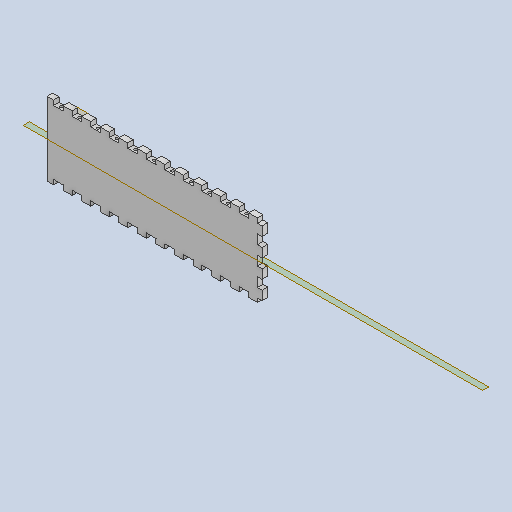
# Autodesk Inventor part: 00_Baseplate_Simmo_side3
Saved by Autodesk Inventor 2022 (Build 260153000, 153)
## iProperties
Created: 2022-04-28
Part Number: 00_Baseplate_Simmo_side3
Material: Generisch
Document SubType Name: Modeling
Designer: diederichbenedict
Density: 1 g/cm^3
Appearance: Vorgabe
Author: diederichbenedict
Autodesk Inventor part; units mm, degrees
ref_plane "YZ Plane" through (0, 0, 0) normal (1, 0, 0) x (0, 1, 0)
ref_plane "XZ Plane" through (0, 0, 0) normal (0, 1, 0) x (-1, 0, 0)
ref_plane "XY Plane" through (0, 0, 0) normal (0, 0, 1) x (1, 0, 0)
ref_plane "Arbeitsebene1" through (0, 0, 0) normal (0, 0, 1) x (1, 0, 0)
sketch "Skizze1" plane through (0, 0, 0) normal (0, 0, 1) x (1, 0, 0)
  line L0 (0, 5) -> (10, 5)
  line L1 (10, 0) -> (0, 0)
  line L2 (10, 0) -> (10, 5)
  line L3 (442.7944, 5) -> (442.7944, 0)
  line L4 (0, -68) -> (10, -68)
  line L5 (0, 5) -> (229.5237, 5)
  line L6 (229.5237, 5) -> (229.5237, -68)
  line L7 (229.5237, -68) -> (0, -68)
  line L8 (0, -68) -> (0, 5)
  line L9 (0, -68) -> (229.5237, -68)
  line L10 (229.5237, -68) -> (229.5237, -74)
  line L11 (229.5237, -74) -> (0, -74)
  line L12 (0, -74) -> (0, -68)
  line L13 (0, 0) -> (0, 5)
  line L14 (238.603, -69) -> (238.603, -74)
  line L15 (230.1, -69) -> (230.1, -74)
  line L16 (230.1, -74) -> (220.1, -74)
  line L17 (229.5237, 0.1) -> (229.5237, 5)
  point P0 (450, -68)
  point P1 (450, 0)
  point P2 (442.7944, 5)
  point P3 (450, -68)
extrude "Extrusion1" add sketch "Skizze1" along normal blind 6
sketch "Skizze2" plane through (0, 0, 0) normal (0, 0, -1) x (1, 0, 0)
  line L0 (20, 0) -> (20, -5) projected
  line L1 (10, -5) -> (10, 0) projected
  line L2 (0, -5) -> (0, 74) projected
  line L3 (9.8, -5) -> (20.2, -5)
  line L4 (20.2, -5) -> (20.2, 0)
  line L5 (20.2, 0) -> (9.8, 0)
  line L6 (9.8, 0) -> (9.8, -5)
  point P0 (0, 0)
  dimension "d6" = 0
  dimension "d17" = 0.2
  dimension "d18" = 0.2
  constraints: 8 end point, 2 parallel, 1 horizontal, 1 perpendicular
  measures "d6" distance from line of L1.end L5
  measures "d17" distance between parallel lines of L4 L0
  measures "d18" distance between parallel lines of L6 L1
extrude "Extrusion2" cut sketch "Skizze2" against normal blind 6
sketch "Skizze3" plane through (20.2, 5, 0) normal (0, 1, 0) x (1, 0, 0)
  line L0 (209.3237, 0) -> (0, 0) projected
  line L1 (-10.4, -6) -> (0, -6) projected
  line L2 (0, 0) -> (0, -6) projected
  circle A0 centre (-5.2, -3) radius 1.5
  line L3 (-10.4, -6) -> (-10.4, 0) projected
  point P0 (-20.2, 0)
  point P1 (4.8, 3)
  point P2 (429.8, 0)
  point P3 (429.8, -6)
  dimension "d16" = 3
  dimension "d19" = 5.2
  constraints: 1 centre point
  measures "d16" diameter of A0
  measures "d19" distance from line of A0.centre L3
hole "Bohrung1" at (15, 5, 3) direction (0, -1, 0) diameter 3 depth 20
pattern_linear "Rechteckige Anordnung1" count 24 spacing 20 along (1, 0, 0) of "Extrusion2", "Bohrung1"
ref_plane "Arbeitsebene2" through (0, -34.5, 0) normal (0, -1, 0) x (1, 0, 0)
mirror "Spiegeln1" about plane through (0, -34.5, 0) normal (0, -1, 0) of "Extrusion2", "Bohrung1", "Rechteckige Anordnung1"
sketch "Skizze4" plane through (0, 5, 6) normal (0, 1, 0) x (1, 0, 0)
  line L0 (9.8356, 19.8689) -> (14.6897, 16.3421) projected
  line L1 (20.45, 24.2705) -> (14.6897, 16.3421) projected
  line L2 (15.5959, 27.7972) -> (20.45, 24.2705) projected
  line L3 (15.5959, 27.7972) -> (9.8356, 19.8689) projected
  line L4 (9.8, 0) -> (0, 0) projected
  line L5 (3, 0) -> (-2.0103, 0)
  line L6 (-2.0103, 0) -> (-2.0103, 6)
  line L7 (-2.0103, 6) -> (3, 6)
  line L8 (3, 6) -> (3, 0)
  line L9 (0, 6) -> (0, 0) projected
  line L10 (2.8165, 0) -> (2.8165, 6)
  point P0 (-2.0103, 2.2794)
  point P1 (0, 6)
  point P2 (0, 0)
  point P3 (0, 0)
  dimension "d25" = 3
  constraints: 10 end point, 2 parallel, 1 horizontal, 1 perpendicular, 1 point on line, 1 vertical, 3 other
  measures "d25" distance between parallel lines of L9 L8
extrude "Extrusion3" cut sketch "Skizze4" against normal through all contours L3 L2 L1 L0 | L4 L9 L7 L10 | L5 L6 L7 L9
sketch "Skizze5" plane through (0, 0, 6) normal (0, 0, 1) x (1, 0, 0)
  line L0 (2.8165, 5) -> (2.8165, -74) projected
  line L1 (2.8165, -74) -> (9.8, -74) projected
  line L2 (9.8, -74) -> (9.8, -69) projected
  line L3 (9.8, -69) -> (20.2, -69) projected
  line L4 (20.2, -69) -> (20.2, -74) projected
  line L5 (20.2, -74) -> (29.8, -74) projected
  line L6 (29.8, -74) -> (29.8, -69) projected
  line L7 (29.8, -69) -> (40.2, -69) projected
  line L8 (40.2, -69) -> (40.2, -74) projected
  line L9 (40.2, -74) -> (49.8, -74) projected
  line L10 (49.8, -74) -> (49.8, -69) projected
  line L11 (49.8, -69) -> (60.2, -69) projected
  line L12 (60.2, -69) -> (60.2, -74) projected
  line L13 (60.2, -74) -> (69.8, -74) projected
  line L14 (69.8, -74) -> (69.8, -69) projected
  line L15 (69.8, -69) -> (80.2, -69) projected
  line L16 (80.2, -69) -> (80.2, -74) projected
  line L17 (80.2, -74) -> (89.8, -74) projected
  line L18 (89.8, -74) -> (89.8, -69) projected
  line L19 (89.8, -69) -> (100.2, -69) projected
  line L20 (100.2, -69) -> (100.2, -74) projected
  line L21 (100.2, -74) -> (109.8, -74) projected
  line L22 (109.8, -74) -> (109.8, -69) projected
  line L23 (109.8, -69) -> (120.2, -69) projected
  line L24 (120.2, -69) -> (120.2, -74) projected
  line L25 (120.2, -74) -> (129.8, -74) projected
  line L26 (129.8, -74) -> (129.8, -69) projected
  line L27 (129.8, -69) -> (140.2, -69) projected
  line L28 (140.2, -69) -> (140.2, -74) projected
  line L29 (140.2, -74) -> (149.8, -74) projected
  line L30 (149.8, -74) -> (149.8, -69) projected
  line L31 (149.8, -69) -> (160.2, -69) projected
  line L32 (160.2, -69) -> (160.2, -74) projected
  line L33 (160.2, -74) -> (169.8, -74) projected
  line L34 (169.8, -74) -> (169.8, -69) projected
  line L35 (169.8, -69) -> (180.2, -69) projected
  line L36 (180.2, -69) -> (180.2, -74) projected
  line L37 (180.2, -74) -> (189.8, -74) projected
  line L38 (189.8, -74) -> (189.8, -69) projected
  line L39 (189.8, -69) -> (200.2, -69) projected
  line L40 (200.2, -69) -> (200.2, -74) projected
  line L41 (200.2, -74) -> (209.8, -74) projected
  line L42 (209.8, -74) -> (209.8, -69) projected
  line L43 (209.8, -69) -> (220.2, -69) projected
  line L44 (220.2, -69) -> (220.2, -74) projected
  line L45 (220.2, -74) -> (229.5237, -74) projected
  line L46 (229.5237, -74) -> (229.5237, 5) projected
  line L47 (229.5237, 5) -> (220.2, 5) projected
  line L48 (220.2, 5) -> (220.2, 0) projected
  line L49 (220.2, 0) -> (209.8, 0) projected
  line L50 (209.8, 0) -> (209.8, 5) projected
  line L51 (209.8, 5) -> (200.2, 5) projected
  line L52 (200.2, 5) -> (200.2, 0) projected
  line L53 (200.2, 0) -> (189.8, 0) projected
  line L54 (189.8, 0) -> (189.8, 5) projected
  line L55 (189.8, 5) -> (180.2, 5) projected
  line L56 (180.2, 5) -> (180.2, 0) projected
  line L57 (180.2, 0) -> (169.8, 0) projected
  line L58 (169.8, 0) -> (169.8, 5) projected
  line L59 (169.8, 5) -> (160.2, 5) projected
  line L60 (160.2, 5) -> (160.2, 0) projected
  line L61 (160.2, 0) -> (149.8, 0) projected
  line L62 (149.8, 0) -> (149.8, 5) projected
  line L63 (149.8, 5) -> (140.2, 5) projected
  line L64 (140.2, 5) -> (140.2, 0) projected
  line L65 (140.2, 0) -> (129.8, 0) projected
  line L66 (129.8, 0) -> (129.8, 5) projected
  line L67 (129.8, 5) -> (120.2, 5) projected
  line L68 (120.2, 5) -> (120.2, 0) projected
  line L69 (120.2, 0) -> (109.8, 0) projected
  line L70 (109.8, 0) -> (109.8, 5) projected
  line L71 (109.8, 5) -> (100.2, 5) projected
  line L72 (100.2, 5) -> (100.2, 0) projected
  line L73 (100.2, 0) -> (89.8, 0) projected
  line L74 (89.8, 0) -> (89.8, 5) projected
  line L75 (89.8, 5) -> (80.2, 5) projected
  line L76 (80.2, 5) -> (80.2, 0) projected
  line L77 (80.2, 0) -> (69.8, 0) projected
  line L78 (69.8, 0) -> (69.8, 5) projected
  line L79 (69.8, 5) -> (60.2, 5) projected
  line L80 (60.2, 5) -> (60.2, 0) projected
  line L81 (60.2, 0) -> (49.8, 0) projected
  line L82 (49.8, 0) -> (49.8, 5) projected
  line L83 (49.8, 5) -> (40.2, 5) projected
  line L84 (40.2, 5) -> (40.2, 0) projected
  line L85 (40.2, 0) -> (29.8, 0) projected
  line L86 (29.8, 0) -> (29.8, 5) projected
  line L87 (29.8, 5) -> (20.2, 5) projected
  line L88 (20.2, 5) -> (20.2, 0) projected
  line L89 (20.2, 0) -> (9.8, 0) projected
  line L90 (9.8, 0) -> (9.8, 5) projected
  line L91 (9.8, 5) -> (2.8165, 5) projected
  line L92 (229.5237, 0) -> (234.5237, 0) construction
  line L93 (234.5237, 0) -> (234.5237, -10) construction
  line L94 (234.5237, -10) -> (229.5237, -10) construction
  line L95 (229.5237, -10) -> (229.5237, 0) construction
  line L96 (229.5237, -74) -> (229.5237, 5) projected
  line L97 (234.5237, -0.1) -> (229.5237, -0.1)
  line L98 (229.5237, -0.1) -> (229.5237, -9.9)
  line L99 (229.5237, -9.9) -> (234.5237, -9.9)
  line L100 (234.5237, -9.9) -> (234.5237, -0.1)
  point P0 (0, 0)
  dimension "d29" = 5
  dimension "d30" = 10
  dimension "d31" = 0.1
  dimension "d32" = 0.1
  constraints: 16 end point, 4 parallel, 3 point on line, 2 horizontal, 2 perpendicular
  measures "d29" distance of L93.end L94.end
  measures "d30" distance of L92.end L93.end
  measures "d31" distance between parallel lines of L92 L97
  measures "d32" distance between parallel lines of L94 L99
extrude "Extrusion4" add sketch "Skizze5" against normal up to surface (6 mm away) contours L97 L100 L99 L46
pattern_linear "Rechteckige Anordnung2" count 4 spacing 20 along (0, -1, 0) of "Extrusion4"
